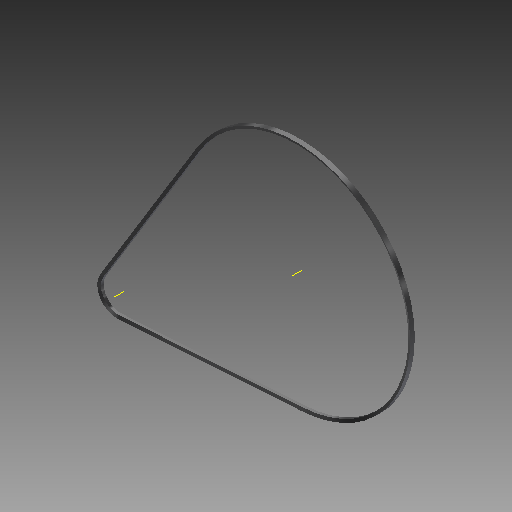
# Autodesk Inventor part: V-Belt
Saved by Autodesk Inventor 2019 (Build 230136000, 136)
## iProperties
Created: 2020-02-18
Part Number: V-Belt
Material: Rubber
Document SubType Name: Modeling
Designer: admin
Density: 0.93 g/cm^3
Appearance: Rubber - Black - Version 1.1
CustomPartVersion: 1
Author: admin
Autodesk Inventor part; units mm, degrees
ref_plane "YZ Plane" through (0, 0, 0) normal (1, 0, 0) x (0, 1, 0)
ref_plane "XZ Plane" through (0, 0, 0) normal (0, 1, 0) x (-1, 0, 0)
sketch "Sketch Path" plane through (0, 0, 0) normal (0, 0, 1) x (1, 0, 0)
  arc A0 (-35.5592, 22.4519) -> (1.1743, -38.3317) centre (-1.4345, 1.5831) ccw
  arc A1 (405.3311, -11.9171) -> (175.7473, 367.9806) centre (389.0265, 237.5507) ccw
  line L0 (405.3311, -11.9171) -> (1.1743, -38.3317)
  line L1 (-35.5592, 22.4519) -> (175.7473, 367.9806)
  constraints: 4 end point, 4 point on circle, 2 centre point
ref_plane "Cross Section Plane" through (1.1743, -38.3317, 0) normal (0.9979, 0.0652, 0) x (0, 0, 1)
sketch "Cross Section" plane through (1.1743, -38.3317, 0) normal (0.9979, 0.0652, 0) x (0, 0, 1)
  line L0 (0, 2.4986) -> (0, -3.5014) construction
  line L1 (-4.25, 0) -> (4.25, 0) construction
  line L2 (-5.1594, 2.4986) -> (5.1594, 2.4986)
  line L3 (5.1594, 2.4986) -> (2.9756, -3.5014)
  line L4 (2.9756, -3.5014) -> (-2.9756, -3.5014)
  line L5 (-2.9756, -3.5014) -> (-5.1594, 2.4986)
  point P0 (0, 0)
  point P1 (0, 0)
  point P2 (0, 0)
  dimension "d0" = 8.5
  dimension "d1" = 2.4986
  dimension "d2" = 40
  dimension "d3" = 6
  constraints: 12 end point, 3 midpoint, 2 parallel, 2 point on line, 1 coincident, 1 perpendicular, 1 vertical, 1 other
  measures "d0" distance of L1.start L1.end
  measures "d1" distance between parallel lines of L2 L1
  measures "d2" angle of L5 L3
  measures "d3" distance between parallel lines of L4 L2
sweep "Belt" add profiles "Cross Section" path "Sketch Path"
equation "\"d0\" = da_Bw"
equation "\"d1\" = da_Hw"
equation "\"d2\" = da_Alfa"
equation "\"d3\" = da_H"
equation "\"da_Alfa\" = 40deg"
equation "\"da_H\" = 6"
equation "\"da_Bw\" = 8.5"
equation "\"da_Hw\" = 2.49859"
body "Solid1"
